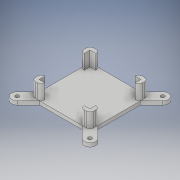
# Autodesk Inventor part: USBHubMount
Saved by Autodesk Inventor 2018 (Build 220112000, 112)
## iProperties
Created: 2019-09-27
Part Number: USBHubMount
Material: Generic
Document SubType Name: Modeling
Designer: anirudh
Density: 1 g/cm^3
Appearance: Default
Author: anirudh
Autodesk Inventor part; units mm, degrees
ref_plane "YZ Plane" through (0, 0, 0) normal (1, 0, 0) x (0, 1, 0)
ref_plane "XZ Plane" through (0, 0, 0) normal (0, 1, 0) x (-1, 0, 0)
ref_plane "XY Plane" through (0, 0, 0) normal (0, 0, 1) x (1, 0, 0)
sketch "Sketch1" plane through (0, 0, 0) normal (0, 1, 0) x (-1, 0, 0)
  line L0 (-24.732, -57.0862) -> (-50.132, -57.0862)
  line L1 (-50.132, -57.0862) -> (-13.2404, -57.0862)
  line L2 (-6.2862, -50.132) -> (-6.2862, -13.2404)
  line L3 (-13.2404, -6.2862) -> (-50.132, -6.2862)
  line L4 (-57.0862, -13.2404) -> (-57.0862, -50.132)
  line L5 (-6.2862, -57.0862) -> (2.6038, -57.0862) construction
  arc A0 (-3.4771, -66.8495) -> (3.4771, -59.8953) centre (0, -63.3724) ccw
  circle A1 centre (0, -63.3724) radius 1.65
  line L6 (-6.2862, -6.2862) -> (2.6038, -6.2862) construction
  line L7 (0, -63.3724) -> (4.9174, -63.3724) construction
  line L8 (-3.4771, -66.8495) -> (-13.2404, -57.0862)
  line L9 (3.4771, -59.8953) -> (-6.2862, -50.132)
  line L10 (-6.2862, -6.2862) -> (2.6038, -6.2862) construction
  line L11 (0, 0) -> (4.9174, 0) construction
  circle A2 centre (0, 0) radius 1.65
  line L12 (-3.4771, 3.4771) -> (-13.2404, -6.2862)
  arc A3 (3.4771, -3.4771) -> (-3.4771, 3.4771) centre (0, 0) ccw
  line L13 (3.4771, -3.4771) -> (-6.2862, -13.2404)
  line L14 (-59.8953, -66.8495) -> (-50.132, -57.0862)
  arc A4 (-66.8495, -59.8953) -> (-59.8953, -66.8495) centre (-63.3724, -63.3724) ccw
  line L15 (-66.8495, -59.8953) -> (-57.0862, -50.132)
  circle A5 centre (-63.3724, -63.3724) radius 1.65
  line L16 (-66.8495, -3.4771) -> (-57.0862, -13.2404)
  arc A6 (-59.8953, 3.4771) -> (-66.8495, -3.4771) centre (-63.3724, 0) ccw
  circle A7 centre (-63.3724, 0) radius 1.65
  line L17 (-59.8953, 3.4771) -> (-50.132, -6.2862)
  dimension "d0" = 25.4
  constraints: 36 end point, 8 centre point, 8 point on circle, 4 coincident, 3 horizontal, 2 parallel, 1 perpendicular
  measures "d0" distance of L0.start L0.end
extrude "Extrusion1" add sketch "Sketch1" along normal blind 3.175
sketch "Sketch2" plane through (0, 3.175, 0) normal (0, 1, 0) x (1, 0, 0)
  line L0 (50.132, 57.0862) -> (13.2404, 57.0862) projected
  line L1 (-3.4771, 59.8953) -> (6.2862, 50.132) projected
  line L2 (13.2404, 57.0862) -> (3.4771, 66.8495) projected
  line L3 (6.2862, 50.132) -> (6.2862, 13.2404) projected
  line L4 (57.0862, 13.2404) -> (57.0862, 50.132) projected
  line L5 (13.2404, 6.2862) -> (50.132, 6.2862) projected
  line L6 (9.4612, 53.9112) -> (9.4612, 48.8312)
  line L7 (9.4612, 48.8312) -> (6.2862, 48.8312)
  line L8 (9.4612, 53.9112) -> (14.5412, 53.9112)
  line L9 (14.5412, 53.9112) -> (14.5412, 57.0862)
  line L10 (6.2862, 48.8312) -> (6.2862, 57.0862)
  line L11 (6.2862, 57.0862) -> (14.5412, 57.0862)
  line L12 (9.4612, 9.4612) -> (9.4612, 14.5412)
  line L13 (9.4612, 14.5412) -> (6.2862, 14.5412)
  line L14 (9.4612, 9.4612) -> (14.5412, 9.4612)
  line L15 (14.5412, 9.4612) -> (14.5412, 6.2862)
  line L16 (13.2404, 6.2862) -> (50.132, 6.2862) projected
  line L17 (14.5412, 6.2862) -> (6.2862, 6.2862)
  line L18 (6.2862, 6.2862) -> (6.2862, 14.5412)
  line L19 (53.9112, 9.4612) -> (48.8312, 9.4612)
  line L20 (48.8312, 9.4612) -> (48.8312, 6.2862)
  line L21 (53.9112, 9.4612) -> (53.9112, 14.5412)
  line L22 (53.9112, 14.5412) -> (57.0862, 14.5412)
  line L23 (48.8312, 6.2862) -> (57.0862, 6.2862)
  line L24 (57.0862, 6.2862) -> (57.0862, 14.5412)
  line L25 (53.9112, 53.9112) -> (48.8312, 53.9112)
  line L26 (48.8312, 53.9112) -> (48.8312, 57.0862)
  line L27 (53.9112, 53.9112) -> (53.9112, 48.8312)
  line L28 (53.9112, 48.8312) -> (57.0862, 48.8312)
  line L29 (57.0862, 48.8312) -> (57.0862, 57.0862)
  line L30 (57.0862, 57.0862) -> (48.8312, 57.0862)
  point P0 (0, 0)
  dimension "d19" = 5.08
  dimension "d20" = 5.08
  dimension "d21" = 5.08
  dimension "d22" = 5.08
  dimension "d23" = 5.08
  dimension "d24" = 5.08
  constraints: 48 end point, 9 perpendicular, 9 point on line, 3 collinear, 2 vertical, 1 horizontal
  measures "d19" distance of L6.start L6.end
  measures "d20" distance of L6.start L8.end
  measures "d21" distance of L12.start L12.end
  measures "d22" distance of L12.start L14.end
  measures "d23" distance of L19.start L19.end
  measures "d24" distance of L19.start L21.end
extrude "Extrusion3" add sketch "Sketch2" along normal blind 12.7 contours L30 L29 L4 L28 L27 L25 L26 L0 | L9 L8 L6 L7 L3 L10 L11 L0 | L4 L24 L23 L5 L20 L19 L21 L22 | L13 L12 L14 L15 L5 L17 L18 L3
fillet "Fillet2" radius 3.175 12 edges at (57.0862, 9.525, -6.2862) (6.2862, 9.525, -6.2862) (57.0862, 9.525, -57.0862) (6.2862, 9.525, -57.0862) (48.8312, 9.525, -6.2862) (57.0862, 9.525, -14.5412) (57.0862, 9.525, -48.8312) (48.8312, 9.525, -57.0862) (14.5412, 9.525, -57.0862) (6.2862, 9.525, -48.8312) (14.5412, 9.525, -6.2862) (6.2862, 9.525, -14.5412)
sketch "Sketch3" plane through (0, 0, 0) normal (0, -1, 0) x (1, 0, 0)
  circle A0 centre (63.3724, 0) radius 1.75
  circle A1 centre (0, 0) radius 1.75
  circle A2 centre (0, -63.3724) radius 1.65 projected
  circle A3 centre (0, -63.3724) radius 1.75
  circle A4 centre (63.3724, -63.3724) radius 1.65 projected
  circle A5 centre (63.3724, -63.3724) radius 1.75
  dimension "d30" = 3.5
  dimension "d31" = 3.5
  dimension "d32" = 3.5
  dimension "d33" = 3.5
  constraints: 4 centre point, 4 coincident
  measures "d30" diameter of A0
  measures "d31" diameter of A1
  measures "d32" diameter of A3
  measures "d33" diameter of A5
body "Solid1"
